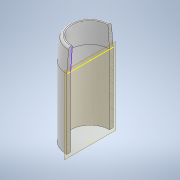
# Autodesk Inventor part: cylinder part
Saved by Autodesk Inventor 2020.2 (Build 242310000, 310)
## iProperties
Created: 2020-09-23
Part Number: cylinder part
Material: Generic
Document SubType Name: Modeling
Designer: Amaan Khalid
Density: 1 g/cm^3
Appearance: Default
Author: Amaan Khalid
Autodesk Inventor part; units mm, degrees
ref_plane "XZ Plane" through (0, 0, 0) normal (0, 1, 0) x (-1, 0, 0)
ref_plane "XY Plane" through (0, 0, 0) normal (0, 0, 1) x (1, 0, 0)
sketch "Sketch1" plane through (0, 0, 0) normal (0, 1, 0) x (-1, 0, 0)
  circle A0 centre (0, 0) radius 13.081
  dimension "d0" = 26.162
  constraints: 1 centre point, 1 coincident
  measures "d0" diameter of A0
extrude "Extrusion1" add sketch "Sketch1" along normal blind 39.37
sketch "Sketch2" plane through (0, 39.37, 0) normal (0, 1, 0) x (1, 0, 0)
  circle A0 centre (0, 0) radius 10.9884
  constraints: 1 centre point, 1 coincident
extrude "Extrusion2" cut sketch "Sketch2" against normal through all
sketch "Sketch3" plane through (0, 39.37, 0) normal (0, 1, 0) x (1, 0, 0)
  point P0 (0, 0)
ref_plane "Work Plane1" through (0, 0, 0) normal (1, 0, 0) x (0, 1, 0)
sketch "Sketch4" plane through (0, 0, 0) normal (1, 0, 0) x (0, 1, 0)
  line L0 (39.37, -13.081) -> (39.37, 13.081) projected
  line L1 (39.37, 13.081) -> (52.07, 13.081) construction
  line L2 (39.37, 0) -> (51.6373, 0)
  line L3 (39.37, 10.9884) -> (39.37, -10.9884) projected
  line L4 (39.37, 10.9884) -> (51.7114, 10.0843)
  line L5 (39.37, 13.081) -> (50.6127, 12.0974)
  line L6 (39.37, 13.081) -> (50.6556, 13.081) construction
  line L7 (51.7671, 10.7215) -> (51.7114, 10.0843)
  arc A0 (51.7671, 10.7215) -> (50.6127, 12.0974) centre (50.502, 10.8322) ccw
  point P0 (0, 0)
  dimension "d6" = 12.7
  dimension "d8" = 5
  dimension "d9" = 1.27
  constraints: 12 end point, 3 horizontal, 2 point on circle, 2 tangent, 1 centre point, 1 equal length, 1 midpoint, 1 perpendicular
  measures "d6" distance of L0.end L4.end
  measures "d8" angle of L5 L6
  measures "d9" radius of A0
revolve "Revolution1" add sketch "Sketch4" angle 360 about axis through (0, 39.37, 0) along (0, 1, 0)
sketch "Sketch5" plane through (0, 0, 0) normal (1, 0, 0) x (0, 1, 0)
  line L0 (39.37, -13.081) -> (39.37, 13.081) projected
  line L1 (39.37, 10.9828) -> (51.7114, 10.0843)
  line L2 (51.7114, 10.0843) -> (39.37, 10.9884) projected
  point P0 (0, 0)
  constraints: 2 end point, 2 point on line
body "Solid1"
